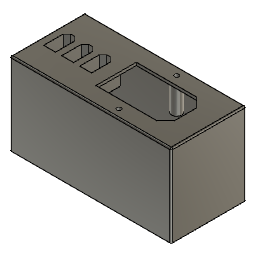
Power supply cover (Autodesk Fusion 360 design; units mm, degrees)
Autodesk Fusion 360 part; units mm, degrees
note: some values were not read from the file. Set by a fixed rule: which sketch regions a step uses.
sketch "Box" plane through (0, 0, 0) normal (0, 0, 1) x (1, 0, 0)
  line L0 (55, 25) -> (-55, 25)
  line L1 (-55, 25) -> (-55, -25)
  line L2 (-55, -25) -> (55, -25)
  line L3 (55, -25) -> (55, 25)
  line L4 (55, 25) -> (-55, -25) construction
  line L5 (-55, 25) -> (55, -25) construction
  line L6 (56, -26) -> (-56, -26)
  line L7 (-56, -26) -> (-56, 26)
  line L8 (-56, 26) -> (56, 26)
  line L9 (56, 26) -> (56, -26)
  line L10 (56, -26) -> (-56, 26) construction
  line L11 (-56, -26) -> (56, 26) construction
  dimension "d2" = 110
  dimension "d3" = 50
  dimension "d4" = 112
  dimension "d5" = 52
  constraint horizontal L0
  constraint perpendicular L0 L1
  constraint parallel L0 L2
  constraint parallel L1 L3
  constraint coincident L4 origin
  constraint coincident L5 origin
  constraint horizontal L6
  constraint perpendicular L6 L7
  constraint parallel L6 L8
  constraint parallel L7 L9
  constraint coincident L10 origin
  constraint coincident L11 origin
  measures "d2" distance of L1.end L2.end
  measures "d3" distance of L0.end L1.end
  measures "d4" distance of L7.end L8.end
  measures "d5" distance of L6.end L7.end
extrude "Extrude1" add sketch "Box" along normal blind 55
fillet "Fillet1" radius 1 4 edges at (56, -26, 27.5) (-56, -26, 27.5) (56, 26, 27.5) (-56, 26, 27.5)
fillet "Fillet2" radius 1 4 edges at (55, -25, 27.5) (55, 25, 27.5) (-55, 25, 27.5) (-55, -25, 27.5)
ref_plane "WorkPlane1" through (0, 0, 55) normal (0, 0, 1) x (1, 0, 0)
sketch "Lid" plane through (0, 0, 55) normal (0, 0, 1) x (1, 0, 0)
  line L0 (55, -26) -> (-55, -26)
  line L1 (-56, -25) -> (-56, 25)
  line L2 (-55, 26) -> (55, 26)
  line L3 (56, 25) -> (56, -25)
  line L4 (56, -26) -> (-56, 26) construction
  line L5 (-56, -26) -> (56, 26) construction
  arc A0 (-55, 26) -> (-56, 25) centre (-55, 25) ccw
  arc A1 (56, 25) -> (55, 26) centre (55, 25) ccw
  arc A2 (55, -26) -> (56, -25) centre (55, -25) ccw
  arc A3 (-56, -25) -> (-55, -26) centre (-55, -25) ccw
  dimension "d13" = 112
  dimension "d14" = 52
  dimension "d15" = 1
  dimension "d16" = 1
  dimension "d17" = 1
  dimension "d18" = 1
  constraint horizontal L0
  constraint perpendicular L0 L1
  constraint parallel L0 L2
  constraint parallel L1 L3
  constraint coincident L4 origin
  constraint coincident L5 origin
  constraint coincident L4.end L1
  constraint coincident L4.end L2
  constraint tangent L1 A0
  constraint tangent L2 A0
  constraint coincident L5.end L2
  constraint coincident L5.end L3
  constraint tangent L2 A1
  constraint tangent L3 A1
  constraint coincident L4.start L3
  constraint coincident L4.start L0
  constraint tangent L3 A2
  constraint tangent L0 A2
  constraint coincident L5.start L1
  constraint coincident L5.start L0
  constraint tangent L1 A3
  constraint tangent L0 A3
  measures "d13" distance of L4.end L5.end
  measures "d14" distance of L5.start L4.end
  measures "d15" radius of A0
  measures "d16" radius of A1
  measures "d17" radius of A2
  measures "d18" radius of A3
extrude "Extrude2" add sketch "Lid" along normal blind 2
fillet "Fillet3" radius 1 8 edges at (0, 26, 57) (-55.7071, 25.7071, 57) (-56, 0, 57) (-55.7071, -25.7071, 57) (0, -26, 57) (55.7071, -25.7071, 57) (56, 0, 57) (55.7071, 25.7071, 57)
sketch "230 plug" plane through (0, 0, 57) normal (0, 0, 1) x (-1, 0, 0)
  line L0 (-55, -25) -> (55, -25)
  line L1 (55, -25) -> (55, 25)
  line L2 (55, 25) -> (-55, 25)
  line L3 (-55, 25) -> (-55, -25)
  line L4 (8.143, -13.9073) -> (-33.857, -13.9073)
  line L5 (-33.857, 14.0927) -> (8.143, 14.0927)
  line L6 (8.143, 14.0927) -> (8.143, -13.9073)
  line L7 (8.143, -13.9073) -> (-33.857, 14.0927) construction
  line L8 (-33.857, -13.9073) -> (8.143, 14.0927) construction
  line L9 (-33.857, 14.0927) -> (-40.2209, 7.7287)
  line L10 (-33.857, 14.0927) -> (-12.0333, 14.0927) construction
  line L11 (-33.857, -13.9073) -> (-40.2209, -7.5434)
  line L12 (-33.857, -13.9073) -> (-12.0333, -13.9073) construction
  line L13 (-40.2209, -7.5434) -> (-40.2209, 7.7287)
  point P0 (-12.857, 0.0927)
  dimension "d32" = 28
  dimension "d33" = 42
  dimension "d34" = 135
  dimension "d35" = 9
  dimension "d36" = 135
  dimension "d37" = 9
  constraint horizontal L4
  constraint parallel L4 L5
  constraint coincident L7 P0
  constraint coincident L8 P0
  constraint horizontal L10
  constraint horizontal L12
  constraint parallel L3 L13
  measures "d32" distance of L4.end L5.start
  measures "d33" distance of L5.start L5.end
  measures "d34" angle of L9 L10
  measures "d35" distance of L5.start L9.end
  measures "d36" angle of L11 L12
  measures "d37" distance of L4.end L11.end
extrude "Extrude3" cut sketch "230 plug" against normal blind 2 contours L4 L5 L6 L9 L11 L13
ref_plane "WorkPlane2" through (0, 0, 55) normal (0, 0, -1) x (-1, 0, 0)
sketch "Screw Holes" plane through (0, 0, 55) normal (0, 0, -1) x (1, 0, 0)
  line L0 (-8.143, 14.0927) -> (-8.143, -13.9073)
  circle A0 centre (13.857, -19.9073) radius 1.5
  line L1 (-8.143, -13.9073) -> (13.857, -13.9073)
  line L2 (13.857, -13.9073) -> (13.857, -19.9073)
  circle A1 centre (13.857, -19.9073) radius 3.5
  line L3 (-8.143, 14.0927) -> (13.857, 14.0927)
  line L4 (13.857, 14.0927) -> (13.857, 20.0927)
  circle A2 centre (13.857, 20.0927) radius 3.5
  circle A3 centre (13.857, 20.0927) radius 1.5
  dimension "d44" = 3
  dimension "d45" = 22
  dimension "d46" = 6
  dimension "d47" = 7
  dimension "d49" = 22
  dimension "d50" = 6
  dimension "d51" = 7
  dimension "d52" = 3
  constraint coincident L0.end L1.start
  constraint perpendicular L0 L1
  constraint perpendicular L1 L2
  constraint coincident A0.centre L2.end
  constraint concentric A0 A1
  constraint coincident L0.start L3.start
  constraint perpendicular L0 L3
  constraint perpendicular L3 L4
  constraint coincident L4.end A2.centre
  constraint concentric A2 A3
  measures "d44" diameter of A0
  measures "d45" distance of L0.end L1.end
  measures "d46" distance of L1.end A0.centre
  measures "d47" diameter of A1
  measures "d49" distance of L0.start L3.end
  measures "d50" distance of L3.end L4.end
  measures "d51" diameter of A2
  measures "d52" diameter of A3
extrude "Extrude5" add sketch "Screw Holes" along normal blind 20
extrude "Extrude6" cut sketch "Screw Holes" against normal blind 2 contours A0 | A3
sketch "XT60 plug 1" plane through (0, 0, 55) normal (0, 0, -1) x (1, 0, 0)
  circle A0 centre (13.857, -19.9073) radius 3.5
  line L0 (40.2209, 7.7287) -> (40.2209, -7.5434)
  line L1 (40.2209, -7.5434) -> (33.857, -13.9073)
  line L2 (33.857, -13.9073) -> (-8.143, -13.9073)
  line L3 (-8.143, -13.9073) -> (-8.143, 14.0927)
  line L4 (-8.143, 14.0927) -> (33.857, 14.0927)
  line L5 (33.857, 14.0927) -> (40.2209, 7.7287)
  arc A1 (-54, 25) -> (-55, 24) centre (-54, 24) ccw
  line L6 (-55, 24) -> (-55, -24)
  arc A2 (-55, -24) -> (-54, -25) centre (-54, -24) ccw
  line L7 (-54, -25) -> (54, -25)
  arc A3 (54, -25) -> (55, -24) centre (54, -24) ccw
  line L8 (55, -24) -> (55, 24)
  arc A4 (55, 24) -> (54, 25) centre (54, 24) ccw
  line L9 (54, 25) -> (-54, 25)
  circle A5 centre (13.857, 20.0927) radius 3.5
  line L10 (-50.4445, 8.0625) -> (-42.2445, 8.0625)
  line L11 (-42.2445, -5.4375) -> (-44.8962, -8.0891)
  line L12 (-50.4445, -5.4375) -> (-47.7929, -8.0891)
  line L13 (-47.7929, -8.0891) -> (-44.8962, -8.0891)
  line L14 (-37.9445, 8.0625) -> (-29.7445, 8.0625)
  line L15 (-29.7445, 8.0625) -> (-29.7445, -5.4375)
  line L16 (-29.7445, -5.4375) -> (-32.3962, -8.0891)
  line L17 (-37.9445, -5.4375) -> (-35.2929, -8.0891)
  line L18 (-35.2929, -8.0891) -> (-32.3962, -8.0891)
  line L19 (-17.2445, 8.0625) -> (-25.4445, 8.0625)
  line L20 (-25.4445, 8.0625) -> (-25.4445, -5.4375)
  line L21 (-25.4445, -5.4375) -> (-22.7929, -8.0891)
  line L22 (-17.2445, -5.4375) -> (-19.8962, -8.0891)
  line L23 (-22.7929, -8.0891) -> (-19.8962, -8.0891)
  line L24 (-42.2445, -5.4375) -> (-42.2445, 8.0625)
  line L25 (-37.9445, -5.4375) -> (-37.9445, 8.0625)
  line L26 (-17.2445, -5.4375) -> (-17.2445, 8.0625)
  line L27 (-50.4445, 8.0625) -> (-50.4445, -5.4375)
  line L28 (-42.2445, 1.3125) -> (-37.9445, 1.3125)
  line L29 (-29.7445, 1.3125) -> (-25.4445, 1.3125)
  dimension "d70" = 3.75
  dimension "d71" = 3.75
  dimension "d72" = 8.2
  dimension "d75" = 3.75
  dimension "d76" = 3.75
  dimension "d79" = 8.2
  dimension "d80" = 13.5
  dimension "d81" = 3.75
  dimension "d83" = 3.75
  dimension "d89" = 8.2
  dimension "d91" = 4.3
  constraint perpendicular L11 L12
  constraint horizontal L13
  constraint perpendicular L14 L15
  constraint perpendicular L16 L17
  constraint perpendicular L15 L19
  constraint perpendicular L16 L21
  constraint horizontal L23
  constraint perpendicular L10 L24
  constraint perpendicular L14 L25
  constraint perpendicular L19 L26
  constraint perpendicular L10 L27
  constraint equal L24 L27
  constraint equal L15 L25
  constraint equal L20 L26
  constraint collinear L10 L14
  constraint collinear L14 L19
  constraint equal L13 L18
  constraint parallel L18 L23
  constraint parallel L15 L20
  constraint midpoint L24 L28.start
  constraint midpoint L25 L28.end
  constraint perpendicular L25 L28
  constraint midpoint L15 L29.start
  constraint perpendicular L15 L29
  constraint coincident L20 L29.end
  constraint equal L28 L29
  constraint collinear L13 L23
  constraint collinear L13 L18
  measures "d70" distance of L11.start L11.end
  measures "d71" distance of L12.start L12.end
  measures "d72" distance of L14.start L14.end
  measures "d75" distance of L15.end L16.end
  measures "d76" distance of L17.start L17.end
  measures "d79" distance of L19.start L19.end
  measures "d80" distance of L19.end L20.end
  measures "d81" distance of L20.end L21.end
  measures "d83" distance of L22.start L22.end
  measures "d89" distance of L10.start L10.end
  measures "d91" distance of L29.start L29.end
extrude "Extrude7" cut sketch "XT60 plug 1" against normal blind 2 contours L10 L11 L12 L13 L24 L27 | L14 L15 L16 L17 L18 L25 | L19 L20 L21 L22 L23 L26
sketch "Sketch7" plane through (0, 0, 55) normal (0, 0, -1) x (1, 0, 0)
  line L0 (-47.7929, -8.0891) -> (-50.4445, -5.4375)
  line L1 (-50.4445, 8.0625) -> (-42.2445, 8.0625)
  line L2 (-42.2445, 8.0625) -> (-42.2445, -5.4375)
  line L3 (-42.2445, -5.4375) -> (-44.8962, -8.0891)
  line L4 (-44.8962, -8.0891) -> (-47.7929, -8.0891)
  line L5 (-29.7445, -5.4375) -> (-32.3962, -8.0891)
  line L6 (-32.3962, -8.0891) -> (-35.2929, -8.0891)
  line L7 (-35.2929, -8.0891) -> (-37.9445, -5.4375)
  line L8 (-37.9445, -5.4375) -> (-37.9445, 8.0625)
  line L9 (-37.9445, 8.0625) -> (-29.7445, 8.0625)
  line L10 (-29.7445, 8.0625) -> (-29.7445, -5.4375)
  line L11 (-25.4445, 8.0625) -> (-17.2445, 8.0625)
  line L12 (-17.2445, 8.0625) -> (-17.2445, -5.4375)
  line L13 (-17.2445, -5.4375) -> (-19.8962, -8.0891)
  line L14 (-19.8962, -8.0891) -> (-22.7929, -8.0891)
  line L15 (-22.7929, -8.0891) -> (-25.4445, -5.4375)
  line L16 (-25.4445, -5.4375) -> (-25.4445, 8.0625)
  circle A0 centre (13.857, -19.9073) radius 3.5
  line L17 (40.2209, 7.7287) -> (40.2209, -7.5434)
  line L18 (40.2209, -7.5434) -> (33.857, -13.9073)
  line L19 (33.857, -13.9073) -> (-8.143, -13.9073)
  line L20 (-8.143, -13.9073) -> (-8.143, 14.0927)
  line L21 (-8.143, 14.0927) -> (33.857, 14.0927)
  line L22 (33.857, 14.0927) -> (40.2209, 7.7287)
  arc A1 (-54, 25) -> (-55, 24) centre (-54, 24) ccw
  line L23 (-55, 24) -> (-55, -24)
  arc A2 (-55, -24) -> (-54, -25) centre (-54, -24) ccw
  line L24 (-54, -25) -> (54, -25)
  arc A3 (54, -25) -> (55, -24) centre (54, -24) ccw
  line L25 (55, -24) -> (55, 24)
  arc A4 (55, 24) -> (54, 25) centre (54, 24) ccw
  line L26 (54, 25) -> (-54, 25)
  circle A5 centre (13.857, 20.0927) radius 3.5
  line L27 (-15.2847, -9.9279) -> (-52.5832, -9.9279)
  line L28 (-52.5832, -9.9279) -> (-52.5832, 10.117)
  line L29 (-52.5832, 10.117) -> (-15.2847, 10.117)
  line L30 (-15.2847, 10.117) -> (-15.2847, -9.9279)
  line L31 (-15.2847, -9.9279) -> (-52.5832, 10.117) construction
  line L32 (-52.5832, -9.9279) -> (-15.2847, 10.117) construction
  line L33 (-50.4445, -5.4375) -> (-50.4445, 8.0625)
  point P0 (-33.934, 0.0945)
  constraint horizontal L27
  constraint perpendicular L27 L28
  constraint parallel L27 L29
  constraint parallel L28 L30
  constraint coincident L31 P0
  constraint coincident L32 P0
extrude "Extrude8" add sketch "Sketch7" along normal blind 14 contours L27 L28 L29 L30
extrude "Extrude4" [suppressed]
named bodies: "Box"
